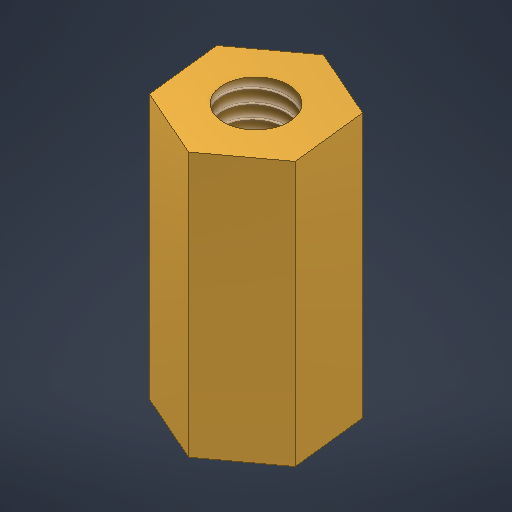
# Autodesk Inventor part: posteNAVIO
Saved by Autodesk Inventor 2026.1 (Build 301233020, 233B)
## iProperties
Created: 2025-10-27
Part Number: posteNAVIO
Material: Latón, amarillo claro
Document SubType Name: Modeling
Designer: rodri
Density: 8.47 g/cm^3
Appearance: Latón - Satinado
Mass: 1.43156 g
Surface Area: 2.8426 cm^2
Volume: 0.169016 cm^3
Author: rodri
Autodesk Inventor part; units mm, degrees
ref_plane "YZ Plane" through (0, 0, 0) normal (1, 0, 0) x (0, 1, 0)
ref_plane "XZ Plane" through (0, 0, 0) normal (0, 1, 0) x (-1, 0, 0)
ref_plane "XY Plane" through (0, 0, 0) normal (0, 0, 1) x (1, 0, 0)
sketch "Boceto1" plane through (0, 0, 0) normal (0, 1, 0) x (-1, 0, 0)
  line L0 (2.6437, -1.1593) -> (0.3178, -2.8692)
  line L1 (0.3178, -2.8692) -> (-2.3259, -1.7099)
  line L2 (-2.3259, -1.7099) -> (-2.6437, 1.1593)
  line L3 (-2.6437, 1.1593) -> (-0.3178, 2.8692)
  line L4 (-0.3178, 2.8692) -> (2.3259, 1.7099)
  line L5 (2.3259, 1.7099) -> (2.6437, -1.1593)
  point P0 (0, 0)
  point P1 (0, 0)
  dimension "d0" = 5
  constraints: 12 end point, 1 coincident, 13 other
  measures "d0" distance between parallel lines of L4 L1
extrude "Extrusión1" add sketch "Boceto1" along normal blind 10
sketch "Boceto2" plane through (0, 10, 0) normal (0, 1, 0) x (1, 0, 0)
  point P0 (0, 0)
  point P1 (0, 0)
  constraints: 1 coincident
hole "Agujero1" at (0, 10, 0) direction (0, -1, 0) diameter 2.459 end through all thread size "M3x0.5" class "6H" standard "ISO Metric profile"
